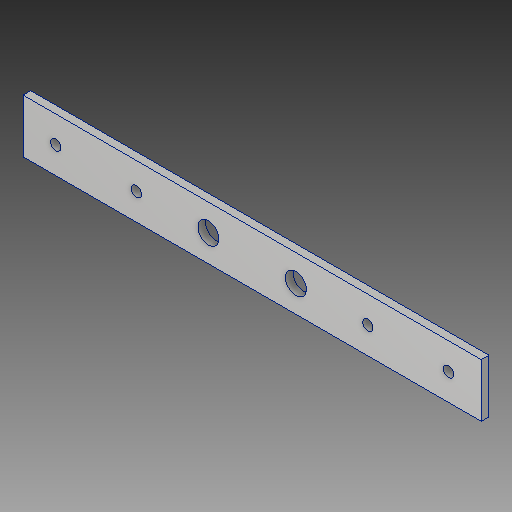
# Autodesk Inventor part: side cutout
Saved by Autodesk Inventor 2017 (Build 210142000, 142)
## iProperties
Created: 2016-10-02
Part Number: side cutout
Material: Aluminum 6061
Document SubType Name: Modeling
Designer: vslabsal
Density: 2.7 g/cm^3
Appearance: Aluminum - Flat
Author: vslabsal
Autodesk Inventor part; units mm, degrees
ref_plane "YZ Plane" through (0, 0, 0) normal (1, 0, 0) x (0, 1, 0)
ref_plane "XZ Plane" through (0, 0, 0) normal (0, 1, 0) x (-1, 0, 0)
ref_plane "XY Plane" through (0, 0, 0) normal (0, 0, 1) x (1, 0, 0)
sketch "Sketch2" plane through (0, 0, 0) normal (0, 0, 1) x (1, 0, 0)
  line L0 (469.9, 22.205) -> (469.9, -34.945)
  line L1 (-99.06, -34.945) -> (-99.06, 22.205)
  circle A0 centre (-58.42, -4.7925) radius 6.35
  circle A1 centre (41.716, -4.7925) radius 6.35
  circle A2 centre (131.092, -4.7925) radius 13
  circle A3 centre (429.26, -4.7925) radius 6.35
  circle A4 centre (329.124, -4.7925) radius 6.35
  circle A5 centre (239.748, -4.7925) radius 13
  line L2 (-99.06, 28.36) -> (469.9, 28.36)
  line L3 (-99.06, -37.945) -> (469.9, -37.945)
  line L4 (-99.06, 22.205) -> (-99.06, 28.36)
  line L5 (-99.06, -37.945) -> (-99.06, -34.945)
  line L6 (469.9, -37.945) -> (469.9, -34.945)
  line L7 (469.9, 22.205) -> (469.9, 28.36)
  point P0 (0, 0)
  point P1 (0, 0)
  dimension "d25" = 12.7
  dimension "d26" = 12.7
  dimension "d27" = 26
  dimension "d28" = 12.7
  dimension "d29" = 12.7
  dimension "d30" = 26
  dimension "d31" = 568.96
  dimension "d32" = 40.64
  dimension "d33" = 140.776
  dimension "d34" = 230.152
  dimension "d35" = 230.152
  dimension "d36" = 40.64
  dimension "d37" = 140.776
  dimension "d38" = 66.305
  dimension "d39" = 33.1525
  dimension "d40" = 33.1525
  dimension "d41" = 33.1525
  dimension "d42" = 33.1525
  dimension "d43" = 33.1525
  dimension "d44" = 33.1525
  constraints: 16 end point, 6 centre point, 2 horizontal, 2 parallel, 1 collinear, 1 perpendicular
  measures "d25" diameter of A0
  measures "d26" diameter of A1
  measures "d27" diameter of A2
  measures "d28" diameter of A3
  measures "d29" diameter of A4
  measures "d30" diameter of A5
  measures "d31" distance between parallel lines of L0 L1
  measures "d32" distance from line of A0.centre L1
  measures "d33" distance from line of A1.centre L1
  measures "d34" distance from line of A2.centre L1
  measures "d35" distance from line of A5.centre L0
  measures "d36" distance from line of A3.centre L0
  measures "d37" distance from line of A4.centre L0
  measures "d38" distance between parallel lines of L2 L3
  measures "d39" distance from line of L3 A0.centre
  measures "d40" distance from line of L3 A1.centre
  measures "d41" distance from line of L3 A2.centre
  measures "d42" distance from line of L3 A5.centre
  measures "d43" distance from line of L3 A4.centre
  measures "d44" distance from line of L3 A3.centre
extrude "Extrusion1" add sketch "Sketch2" along normal blind 9.525
body "Solid1"
